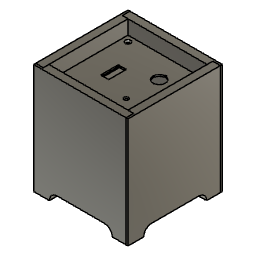
box (Autodesk Fusion 360 design; units mm, degrees)
Autodesk Fusion 360 part; units mm, degrees
sketch "base sketch" plane through (0, 0, 0) normal (0, 0, 1) x (1, 0, 0)
  line L0 (76.2, 76.2) -> (-76.2, 76.2)
  line L1 (-76.2, 76.2) -> (-76.2, -76.2)
  line L2 (-76.2, -76.2) -> (76.2, -76.2)
  line L3 (76.2, -76.2) -> (76.2, 76.2)
  line L4 (76.2, 76.2) -> (-76.2, -76.2) construction
  line L5 (-76.2, 76.2) -> (76.2, -76.2) construction
  line L6 (-76.2, -73.025) -> (-63.9, -73.025)
  line L7 (-63.9, -73.025) -> (-63.9, -63.9)
  line L8 (-63.9, -63.9) -> (73.025, -63.9)
  line L9 (73.025, -63.9) -> (73.025, -76.2)
  dimension "d1" = 152.4
  dimension "d2" = 152.4
  dimension "ply" = 12.3
  dimension "d4" = 12.3
  dimension "outside_radius" = 3.175
  dimension "d6" = 3.175
  constraint horizontal L0
  constraint perpendicular L0 L1
  constraint parallel L0 L2
  constraint parallel L1 L3
  constraint coincident L4 origin
  constraint coincident L5 origin
  constraint coincident L1 L6.start
  constraint perpendicular L1 L6
  constraint perpendicular L6 L7
  constraint coincident L2 L9.end
  constraint perpendicular L2 L9
  constraint horizontal L8
  measures "d1" distance of L1.end L2.end
  measures "d2" distance of L0.end L1.end
  measures "ply" distance of L2 L8
  measures "d4" distance of L1 L7
  measures "outside_radius" distance of L2 L6
  measures "d6" distance of L3 L9
extrude "Extrude1" add sketch "base sketch" along normal blind 177.8 contours L1 L2 L6 L7 L8 L9 makes body 1 in component "side"
sketch "bottom gap" plane through (0, -76.2, 0) normal (0, -1, 0) x (1, 0, 0) in component "side"
  line L0 (-76.2, 0) -> (73.025, 0)
  line L1 (73.025, 0) -> (73.025, 177.8)
  line L2 (73.025, 177.8) -> (-76.2, 177.8)
  line L3 (-76.2, 177.8) -> (-76.2, 0)
  line L4 (-76.2, 0) -> (-78.2761, 0) construction
  line L5 (76.2, 0) -> (-76.2, 0)
  line L6 (76.2, 0) -> (-76.2, 0) construction
  line L7 (0, 0) -> (0, 12.7) construction
  line L8 (-38.1, 12.7) -> (38.1, 12.7)
  arc A0 (-38.1, 12.7) -> (-50.8, 0) centre (-38.1, 0) ccw
  line L9 (-76.2, 0) -> (76.2, 0)
  arc A1 (50.8, 0) -> (38.1, 12.7) centre (38.1, 0) ccw
  point P0 (76.2, 0)
  dimension "d9" = 12.7
  dimension "d10" = 25.4
  dimension "d12" = 25.4
  constraint coincident L0.start L3.end
  constraint coincident P0 L5.start
  constraint coincident L7.start origin
  constraint perpendicular L5 L7
  constraint horizontal L8
  constraint coincident L7.end L8
  constraint coincident L5 A0.centre
  constraint tangent L8 A0
  constraint coincident A0.end L9
  constraint coincident L9 A1.start
  constraint coincident L5 A1.centre
  constraint coincident L8.end A1.end
  constraint tangent L8 A1
  measures "d9" distance of L6 L8
  measures "d10" distance of L0.start A0.end
  measures "d12" distance of P0 A1.start
extrude "Extrude2" cut sketch "bottom gap" against normal up to surface (12.3 mm away) contours L0 L5 L8 A0 L9 A1 bodies 1 in component "side"
component_pattern "component pattern"
ref_plane "WorkPlane1" through (0, 0, 25.4) normal (0, 0, 1) x (1, 0, 0)
sketch "Sketch3" plane through (0, 0, 25.4) normal (0, 0, 1) x (1, 0, 0)
  circle A0 centre (55.4048, 55.4048) radius 6.1
  line L0 (76.2, 76.2) -> (-76.2, -76.2)
  line L1 (-73.025, 63.9) -> (63.9, 63.9) construction
  line L2 (63.9, 73.025) -> (63.9, -63.9) construction
  line L3 (-63.9, -73.025) -> (-63.9, 63.9)
  line L4 (-38.1, 63.9) -> (38.1, 63.9)
  line L5 (76.2, 73.025) -> (76.2, 76.2)
  line L6 (76.2, 76.2) -> (-73.025, 76.2)
  line L7 (-73.025, 76.2) -> (-73.025, 63.9)
  line L8 (-73.025, 63.9) -> (63.9, 63.9)
  line L9 (63.9, 63.9) -> (63.9, 73.025)
  line L10 (63.9, 73.025) -> (76.2, 73.025)
  line L11 (-73.025, 76.2) -> (-76.2, 76.2)
  line L12 (-76.2, 76.2) -> (-76.2, -73.025)
  line L13 (-76.2, -73.025) -> (-63.9, -73.025)
  line L14 (-63.9, -73.025) -> (-63.9, 63.9)
  line L15 (-63.9, 63.9) -> (-73.025, 63.9)
  line L16 (-73.025, 63.9) -> (-73.025, 76.2)
  line L17 (-76.2, -73.025) -> (-76.2, -76.2)
  line L18 (-76.2, -76.2) -> (73.025, -76.2)
  line L19 (73.025, -76.2) -> (73.025, -63.9)
  line L20 (73.025, -63.9) -> (-63.9, -63.9)
  line L21 (-63.9, -63.9) -> (-63.9, -73.025)
  line L22 (-63.9, -73.025) -> (-76.2, -73.025)
  line L23 (73.025, -76.2) -> (76.2, -76.2)
  line L24 (76.2, -76.2) -> (76.2, 73.025)
  line L25 (76.2, 73.025) -> (63.9, 73.025)
  line L26 (63.9, 73.025) -> (63.9, -63.9)
  line L27 (63.9, -63.9) -> (73.025, -63.9)
  line L28 (73.025, -63.9) -> (73.025, -76.2)
  line L29 (-68, 68) -> (68, 68)
  line L30 (68, 68) -> (68, -68)
  line L31 (68, -68) -> (-68, -68)
  line L32 (-68, -68) -> (-68, 68)
  line L33 (-63.9, -63.9) -> (73.025, -63.9)
  line L34 (61.85, 36.85) -> (61.85, -36.85)
  line L35 (36.85, -61.85) -> (-36.85, -61.85)
  line L36 (-61.85, -36.85) -> (-61.85, 36.85)
  line L37 (-36.85, 61.85) -> (36.85, 61.85)
  line L38 (-36.85, -61.85) -> (-61.85, -36.85)
  line L39 (61.85, -36.85) -> (36.85, -61.85)
  line L40 (-61.85, 36.85) -> (-36.85, 61.85)
  line L41 (61.85, 36.85) -> (36.85, 61.85)
  point P0 (61.85, 61.85)
  point P1 (61.85, -61.85)
  point P2 (-61.85, -61.85)
  point P3 (-61.85, 61.85)
  dimension "d18" = 12.2
  dimension "d27" = 4.1
  dimension "d28" = 4.1
  dimension "d29" = 4.1
  dimension "d30" = 4.1
  dimension "d32" = 25
  dimension "d33" = 25
  dimension "d34" = 25
  dimension "d35" = 25
  dimension "d36" = 25
  dimension "d37" = 25
  dimension "d38" = 25
  dimension "d39" = 25
  constraint coincident A0.centre L0
  constraint horizontal L29
  constraint vertical L30
  constraint horizontal L31
  constraint vertical L32
  constraint coincident P2 L35
  constraint coincident P2 L36
  constraint coincident P1 L34
  constraint coincident P1 L35
  constraint coincident P3 L36
  constraint coincident P3 L37
  constraint coincident P0 L34
  constraint coincident P0 L37
  measures "d18" diameter of A0
  measures "d27" distance of L8 L29
  measures "d28" distance of L14 L32
  measures "d29" distance of L31 L33
  measures "d30" distance of L26 L30
  measures "d32" distance of P2 L35.end
  measures "d33" distance of P2 L36.start
  measures "d34" distance of P1 L34.end
  measures "d35" distance of P1 L35.start
  measures "d36" distance of P3 L36.end
  measures "d37" distance of P3 L37.start
  measures "d38" distance of P0 L34.start
  measures "d39" distance of P0 L37.end
extrude "Extrude1'" add sketch "Sketch3" along normal blind 12.3 separate body contours A0 L0 | A0 L0 L20 L26 L33 L34 L35 L38 L39 L41 | A0 L0 | A0 L0 L3 L4 L8 L14 L36 L37 L38 L40 L41 | L0 L9 L26 L29 | L4 L8 L9 L15 L26 L29 L32 | L0 L20 L26 L27 L30 L33 | L3 L14 L20 L21 L27 L30 L31 L33 | L0 L3 L14 L21 L31 | L0 L3 L8 L14 L15 L32 makes body 2 in component "bottom"
sketch "Sketch1" plane through (73.025, 0, 0) normal (1, 0, 0) x (0, 1, 0) in component "side"
  line L0 (-76.2, 0) -> (-63.9, 0)
  line L1 (-63.9, 0) -> (-63.9, 177.8)
  line L2 (-63.9, 177.8) -> (-76.2, 177.8)
  line L3 (-76.2, 177.8) -> (-76.2, 0)
  line L4 (-68, 25.4) -> (68, 25.4)
  line L5 (68, 25.4) -> (68, 37.7)
  line L6 (68, 37.7) -> (-68, 37.7)
  line L7 (-68, 37.7) -> (-68, 25.4)
  line L8 (-68, 140.4) -> (68, 140.4)
  line L9 (68, 140.4) -> (68, 152.7)
  line L10 (68, 152.7) -> (-68, 152.7)
  line L11 (-68, 152.7) -> (-68, 140.4)
extrude "Extrude3" cut sketch "Sketch1" against normal up to surface (136.925 mm away) contours L1 L4 L6 L7 | L1 L8 L10 L11 bodies 1 in component "side"
extrude "Extrude1''" add sketch "Sketch3" along normal blind 12.3 separate body contours A0 L0 | A0 L0 L20 L26 L33 L34 L35 L38 L39 L41 | A0 L0 | A0 L0 L3 L4 L8 L14 L36 L37 L38 L40 L41 | L0 L9 L26 L29 | L4 L8 L9 L15 L26 L29 L32 | L0 L20 L26 L27 L30 L33 | L3 L14 L20 L21 L27 L30 L31 L33 | L0 L3 L14 L21 L31 | L0 L3 L8 L14 L15 L32 makes body 3 in component "top"
extrude "Extrude2'" cut sketch "Sketch3" along normal blind 2.75 contours A0 L0 | A0 L0 bodies 2 in component "bottom"
pattern_circular "C-Pattern1" count 4 over 360 about axis through (0, 0, 1.75) along (0, 0, 1) of "Extrude2'" in component "bottom"
extrude "Extrude1'''" add sketch "base sketch" along normal blind 177.8 separate body contours L1 L2 L6 L7 L8 L9 makes body 4 in component "side sensor"
sketch "bottom gap (2)" plane through (0, -76.2, 0) normal (0, -1, 0) x (1, 0, 0) in component "side sensor"
  line L0 (-76.2, 0) -> (73.025, 0)
  line L1 (73.025, 0) -> (73.025, 177.8)
  line L2 (73.025, 177.8) -> (-76.2, 177.8)
  line L3 (-76.2, 177.8) -> (-76.2, 0)
  line L4 (-76.2, 0) -> (-78.2761, 0) construction
  line L5 (76.2, 0) -> (-76.2, 0)
  line L6 (76.2, 0) -> (-76.2, 0) construction
  line L7 (0, 0) -> (0, 12.7) construction
  line L8 (-38.1, 12.7) -> (38.1, 12.7)
  arc A0 (-38.1, 12.7) -> (-50.8, 0) centre (-38.1, 0) ccw
  line L9 (-76.2, 0) -> (76.2, 0)
  arc A1 (50.8, 0) -> (38.1, 12.7) centre (38.1, 0) ccw
  point P0 (76.2, 0)
  dimension "d9_1" = 12.7
  dimension "d10_1" = 25.4
  dimension "d12_1" = 25.4
  constraint coincident L0.start L3.end
  constraint coincident P0 L5.start
  constraint coincident L7.start origin
  constraint perpendicular L5 L7
  constraint horizontal L8
  constraint coincident L7.end L8
  constraint coincident L5 A0.centre
  constraint tangent L8 A0
  constraint coincident A0.end L9
  constraint coincident L9 A1.start
  constraint coincident L5 A1.centre
  constraint coincident L8.end A1.end
  constraint tangent L8 A1
  measures "d9_1" distance of L6 L8
  measures "d10_1" distance of L0.start A0.end
  measures "d12_1" distance of P0 A1.start
extrude "Extrude2''" cut sketch "bottom gap (2)" against normal up to surface (12.3 mm away) contours L0 L5 L8 A0 L9 A1 bodies 4 in component "side sensor"
sketch "Sketch1 (2)" plane through (73.025, 0, 0) normal (1, 0, 0) x (0, 1, 0) in component "side sensor"
  line L0 (-76.2, 0) -> (-63.9, 0)
  line L1 (-63.9, 0) -> (-63.9, 177.8)
  line L2 (-63.9, 177.8) -> (-76.2, 177.8)
  line L3 (-76.2, 177.8) -> (-76.2, 0)
  line L4 (-68, 25.4) -> (68, 25.4)
  line L5 (68, 25.4) -> (68, 37.7)
  line L6 (68, 37.7) -> (-68, 37.7)
  line L7 (-68, 37.7) -> (-68, 25.4)
  line L8 (-68, 140.4) -> (68, 140.4)
  line L9 (68, 140.4) -> (68, 152.7)
  line L10 (68, 152.7) -> (-68, 152.7)
  line L11 (-68, 152.7) -> (-68, 140.4)
extrude "Extrude3'" cut sketch "Sketch1 (2)" against normal up to surface (136.925 mm away) contours L1 L4 L6 L7 | L1 L8 L10 L11 bodies 4 in component "side sensor"
sketch "sensor" plane through (-76.2, 0, 0) normal (-1, 0, 0) x (0, -1, 0)
  arc A0 (50.8, 0) -> (38.1, 12.7) centre (38.1, 0) ccw
  line L0 (50.8, 0) -> (73.025, 0)
  line L1 (73.025, 0) -> (73.025, 177.8)
  line L2 (73.025, 177.8) -> (-76.2, 177.8)
  line L3 (-76.2, 177.8) -> (-76.2, 0)
  line L4 (-76.2, 0) -> (-50.8, 0)
  arc A1 (-38.1, 12.7) -> (-50.8, 0) centre (-38.1, 0) ccw
  line L5 (-38.1, 12.7) -> (38.1, 12.7)
  line L6 (76.2, 0) -> (76.2, 177.8) construction
  line L7 (76.2, 127) -> (-76.2, 127) construction
  line L8 (0, 127) -> (0, 102.1177) construction
  circle A2 centre (-13, 127) radius 8
  circle A3 centre (13, 127) radius 8
  dimension "d48" = 127
  dimension "d49" = 26
  dimension "d50" = 16
  constraint coincident L6 L7.start
  constraint coincident L3 L7.end
  constraint perpendicular L3 L7
  constraint midpoint L7 L8.start
  constraint perpendicular L7 L8
  constraint coincident L7 A2.centre
  constraint coincident L7 A3.centre
  constraint equal A2 A3
  constraint symmetric L8 A2.centre A3.centre
  measures "d48" distance of L0 L7
  measures "d49" distance of A2.centre A3.centre
  measures "d50" diameter of A2
extrude "Extrude4" cut sketch "sensor" against normal up to surface (12.3 mm away) contours A2 | A3 sketch seen with x (0, 1, 0) y (-1, 0, 0) z (0, 0, 1) at (0, 0, 0) bodies 4 in component "side sensor"
sketch "Sketch1 (3)" plane through (0, 0, 25.4) normal (0, 0, -1) x (1, 0, 0) in component "bottom cover"
  circle A0 centre (55.4048, 55.4048) radius 6.1
  circle A1 centre (-55.4048, 55.4048) radius 6.1
  circle A2 centre (-55.4048, -55.4048) radius 6.1
  circle A3 centre (55.4048, -55.4048) radius 6.1
  line L0 (61.85, 36.85) -> (61.85, -36.85)
  line L1 (61.85, -36.85) -> (36.85, -61.85)
  line L2 (36.85, -61.85) -> (-36.85, -61.85)
  line L3 (-36.85, -61.85) -> (-61.85, -36.85)
  line L4 (-61.85, -36.85) -> (-61.85, 36.85)
  line L5 (-61.85, 36.85) -> (-36.85, 61.85)
  line L6 (-36.85, 61.85) -> (36.85, 61.85)
  line L7 (36.85, 61.85) -> (61.85, 36.85)
  line L8 (68, 68) -> (-68, 68)
  line L9 (-68, 68) -> (-68, -68)
  line L10 (-68, -68) -> (68, -68)
  line L11 (68, -68) -> (68, 68)
  line L12 (-62.9, 62.9) -> (62.9, 62.9)
  line L13 (62.9, 62.9) -> (62.9, -62.9)
  line L14 (62.9, -62.9) -> (-62.9, -62.9)
  line L15 (-62.9, -62.9) -> (-62.9, 62.9)
  line L16 (63.9, -38.1) -> (63.9, 38.1)
  line L17 (38.1, 63.9) -> (-38.1, 63.9)
  line L18 (-63.9, 38.1) -> (-63.9, -38.1)
  line L19 (-38.1, -63.9) -> (38.1, -63.9)
  line L20 (0, 0) -> (47.1189, 0) construction
  line L21 (0, 0) -> (0, 34.7733) construction
  circle A4 centre (10, 0) radius 11
  circle A5 centre (-10, 0) radius 11
  line L22 (-10, 11) -> (10, 11)
  line L23 (10, -11) -> (-10, -11)
  line L24 (0, 0) -> (-38.8885, 0) construction
  line L25 (-10, 11) -> (-10, -11)
  line L26 (10, -11) -> (10, 11)
  dimension "d53" = 1
  dimension "d54" = 1
  dimension "d55" = 1
  dimension "d56" = 1
  dimension "d57" = 22
  dimension "d58" = 22
  dimension "d59" = 20
  constraint horizontal L12
  constraint vertical L13
  constraint horizontal L14
  constraint vertical L15
  constraint coincident L20.start L21.start
  constraint horizontal L20
  constraint perpendicular L20 L21
  constraint coincident L20 A4.centre
  constraint coincident A5 L22.start
  constraint coincident A4 L22.end
  constraint tangent A4 L22
  constraint coincident A4 L23.start
  constraint coincident A5 L23.end
  constraint tangent A5 L23
  constraint tangent A4 L23
  constraint tangent A5 L22
  constraint perpendicular L21 L24
  constraint coincident A5.centre L24
  constraint symmetric L21 A4.centre A5.centre
  measures "d53" distance of L13 L16
  measures "d54" distance of L12 L17
  measures "d55" distance of L15 L18
  measures "d56" distance of L14 L19
  measures "d57" diameter of A4
  measures "d58" diameter of A5
  measures "d59" distance of L25 L26
extrude "Extrude1''''" add sketch "Sketch1 (3)" along normal blind 5 separate body contours A0 | A1 | A2 | A3 | L0 L1 L2 L3 L4 L5 L6 L7 | L12 L13 L14 L15 | A4 L26 | A4 A5 L26 | A4 A5 L22 | A4 A5 L23 | A4 A5 | A4 A5 L25 | A5 L25 makes body 5 in component "bottom cover"
extrude "Extrude2'''" cut sketch "Sketch1 (3)" along normal blind 2.7 contours A0 | A1 | A2 | A3 | L0 L1 L2 L3 L4 L5 L6 L7 | A4 L26 | A4 A5 L26 | A4 A5 L22 | A4 A5 L23 | A4 A5 | A4 A5 L25 | A5 L25 bodies 5 in component "bottom cover"
extrude "Extrude1'''''" [suppressed]
extrude "Extrude3''" cut sketch "Sketch1 (3)" along normal blind 30 contours A4 L26 | A5 L25 bodies 5 in component "bottom cover"
extrude "Extrude4'" add sketch "Sketch1 (3)" against normal blind 3 from surface at 2.7 contours A4 A5 L26 | A4 A5 L22 | A4 A5 L23 | A4 A5 | A4 A5 L25 bodies 5 in component "bottom cover"
sketch "Sketch2" plane through (0, 0, 37.7) normal (0, 0, 1) x (-1, 0, 0) in component "top"
  line L0 (-61.85, -36.85) -> (-61.85, 36.85)
  line L1 (-61.85, 36.85) -> (-36.85, 61.85)
  line L2 (-36.85, 61.85) -> (36.85, 61.85)
  line L3 (36.85, 61.85) -> (61.85, 36.85)
  line L4 (61.85, 36.85) -> (61.85, -36.85)
  line L5 (61.85, -36.85) -> (36.85, -61.85)
  line L6 (36.85, -61.85) -> (-36.85, -61.85)
  line L7 (-36.85, -61.85) -> (-61.85, -36.85)
  line L8 (68, 68) -> (-68, 68)
  line L9 (-68, 68) -> (-68, -68)
  line L10 (-68, -68) -> (68, -68)
  line L11 (68, -68) -> (68, 68)
  line L12 (62.9, -62.9) -> (62.9, 62.9) construction
  line L13 (-62.9, -62.9) -> (62.9, -62.9) construction
  line L14 (-62.9, 62.9) -> (-62.9, -62.9) construction
  line L15 (62.9, 62.9) -> (-62.9, 62.9) construction
  line L16 (-61.85, 36.85) -> (-36.85, 61.85)
  line L17 (-36.85, -61.85) -> (-61.85, -36.85)
  line L18 (61.85, -36.85) -> (36.85, -61.85)
  line L19 (36.85, 61.85) -> (61.85, 36.85)
  line L20 (62.9, 62.9) -> (49.35, 49.35) construction
  line L21 (-63.65, -63.65) -> (63.65, -63.65)
  line L22 (63.65, -63.65) -> (63.65, 63.65)
  line L23 (63.65, 63.65) -> (-63.65, 63.65)
  line L24 (-63.65, 63.65) -> (-63.65, -63.65)
  point P0 (54.2997, 54.2997)
  dimension "d71" = 7
  dimension "d72" = 0.75
  constraint coincident L12.end L15.start
  constraint midpoint L19 L20.end
  constraint coincident L20 P0
  measures "d71" distance of L20.end P0
extrude "Extrude1''''''" add sketch "Sketch2" along normal blind 2.5 separate body contours L0 L1 L2 L3 L4 L5 L6 L7 L16 L17 L18 L19 | L21 L22 L23 L24 sketch seen with x (1, 0, 0) y (0, 1, 0) z (0, 0, 1) at (0, 0, 115) makes body 6 in component "top cover"
sketch "Sketch1 (4)" plane through (0, 0, 155.2) normal (0, 0, 1) x (-1, 0, 0) in component "top cover"
  line L0 (-63.65, 63.65) -> (-63.65, -63.65)
  line L1 (-63.65, -63.65) -> (63.65, -63.65)
  line L2 (63.65, -63.65) -> (63.65, 63.65)
  line L3 (63.65, 63.65) -> (-63.65, 63.65)
  point P0 (54.2997, 54.2997)
hole "Hole1" at (-54.2997, -54.2997, 155.2) direction (0, 0, -1) diameter 4.5 depth 10 tip angle 180 countersink diameter 9 countersink angle 90 bodies 6 in component "top cover"
pattern_circular "C-Pattern1'" count 4 over 360 about axis through (0, 0, 1.75) along (0, 0, 1) of "Hole1" in component "top cover"
sketch "Sketch2 (2)" plane through (0, 0, 155.2) normal (0, 0, 1) x (-1, 0, 0) in component "top cover"
  circle A0 centre (54.2997, -54.2997) radius 4.5
  circle A1 centre (-54.2997, -54.2997) radius 4.5
  circle A2 centre (-54.2997, 54.2997) radius 4.5
  circle A3 centre (54.2997, 54.2997) radius 4.5
  line L0 (-63.65, 63.65) -> (-63.65, -63.65)
  line L1 (-63.65, -63.65) -> (63.65, -63.65)
  line L2 (63.65, -63.65) -> (63.65, 63.65)
  line L3 (63.65, 63.65) -> (-63.65, 63.65)
  line L4 (28.7361, 13) -> (18.2361, 13)
  line L5 (18.2361, 13) -> (18.2361, -13)
  line L6 (18.2361, -13) -> (28.7361, -13)
  line L7 (28.7361, -13) -> (28.7361, 13)
  circle A4 centre (-23.7665, 26.567) radius 3.6
  circle A5 centre (-23.7665, -26.567) radius 10
  line L8 (0, 0) -> (54.4333, 0) construction
  circle A6 centre (-23.7665, 26.567) radius 7.5
  line L9 (-23.7665, 26.567) -> (-23.7665, -26.567) construction
  line L10 (29.7361, 19.5) -> (17.2361, 19.5)
  line L11 (17.2361, 19.5) -> (17.2361, -20.5)
  line L12 (17.2361, -20.5) -> (29.7361, -20.5)
  line L13 (29.7361, -20.5) -> (29.7361, 19.5)
  line L14 (23.4861, 13) -> (23.4861, -13) construction
  line L15 (-23.7665, -26.567) -> (-23.7665, -37.6539) construction
  line L16 (-22.2665, -36.4539) -> (-22.2665, -37.6539)
  line L17 (-22.2665, -37.6539) -> (-25.2665, -37.6539)
  line L18 (-25.2665, -37.6539) -> (-25.2665, -36.4539)
  dimension "d82" = 26
  dimension "d83" = 10.5
  dimension "d84" = 7.2
  dimension "d85" = 15
  dimension "d86" = 20
  dimension "d87" = 12.5
  dimension "d88" = 40
  dimension "d89" = 6.5
  dimension "d90" = 1.2
  dimension "d91" = 3
  constraint horizontal L4
  constraint vertical L5
  constraint horizontal L6
  constraint vertical L7
  constraint coincident L8.start origin
  constraint perpendicular L7 L8
  constraint symmetric L4 L6 L8
  constraint concentric A4 A6
  constraint coincident A4.centre A6.centre
  constraint coincident A5.centre L9.end
  constraint vertical L9
  constraint symmetric A5.centre L8 A4.centre
  constraint horizontal L10
  constraint vertical L11
  constraint horizontal L12
  constraint vertical L13
  constraint midpoint L4 L14.start
  constraint midpoint L6 L14.end
  constraint symmetric L11 L13 L14
  constraint parallel L9 L15
  constraint coincident A5 L16.start
  constraint vertical L16
  constraint perpendicular L15 L17
  constraint coincident A5 L18.end
  constraint perpendicular L17 L18
  constraint coincident L15.end L17
  measures "d82" distance of L4 L6
  measures "d83" distance of L5 L7
  measures "d84" diameter of A4
  measures "d85" diameter of A6
  measures "d86" diameter of A5
  measures "d87" distance of L11 L13
  measures "d88" distance of L10 L12
  measures "d89" distance of L4 L10
  measures "d90" distance of L16.start L16.end
  measures "d91" distance of L16.end L17.end
extrude "Extrude2''''" cut sketch "Sketch2 (2)" against normal blind 10 contours L4 L5 L6 L7 | A4 | A5 | A5 L16 L17 L18 bodies 6 in component "top cover"
chamfer "Chamfer1" distance 1.25 angle 45 4 edges at (-28.7361, 0, 155.2) (-23.4861, -13, 155.2) (-18.2361, 0, 155.2) (-23.4861, 13, 155.2) on bodies 6 in component "top cover"
extrude "Extrude3'''" cut sketch "Sketch2 (2)" along normal blind 1 from surface at -2.5 contours L10 L11 L12 L13 bodies 6 in component "top cover"
sketch "Sketch3 (2)" plane through (0, 0, 152.7) normal (0, 0, -1) x (1, 0, 0) in component "top cover"
  line L0 (-29.7361, -20.5) -> (-29.7361, 19.5)
  line L1 (-29.7361, 19.5) -> (-17.2361, 19.5)
  line L2 (-17.2361, 19.5) -> (-17.2361, -20.5)
  line L3 (-17.2361, -20.5) -> (-29.7361, -20.5)
  circle A0 centre (23.7665, 26.567) radius 3.6
  line L4 (25.2665, -36.4539) -> (25.2665, -37.6539)
  line L5 (25.2665, -37.6539) -> (22.2665, -37.6539)
  line L6 (22.2665, -37.6539) -> (22.2665, -36.4539)
  arc A1 (25.2665, -36.4539) -> (22.2665, -36.4539) centre (23.7665, -26.567) ccw
  circle A2 centre (-54.2997, -54.2997) radius 2.25
  circle A3 centre (54.2997, -54.2997) radius 2.25
  circle A4 centre (54.2997, 54.2997) radius 2.25
  circle A5 centre (-54.2997, 54.2997) radius 2.25
  line L7 (63.65, -63.65) -> (63.65, 63.65)
  line L8 (63.65, 63.65) -> (-63.65, 63.65)
  line L9 (-63.65, 63.65) -> (-63.65, -63.65)
  line L10 (-63.65, -63.65) -> (63.65, -63.65)
  line L11 (-31.7361, -22.5) -> (-31.7361, 21.5)
  line L12 (-31.7361, 21.5) -> (-15.2361, 21.5)
  line L13 (-15.2361, 21.5) -> (-15.2361, -22.5)
  line L14 (-15.2361, -22.5) -> (-31.7361, -22.5)
  dimension "d98" = -2
extrude "Extrude4''" add sketch "Sketch3 (2)" along normal blind 2 contours L11 L12 L13 L14 bodies 6 in component "top cover"
component "side" placed x (1, 0, 0) y (0, 1, 0) z (0, 0, 1) at (0, 0, 0)
component "side" placed x (0, 1, 0) y (-1, 0, 0) z (0, 0, 1) at (0, 0, 0)
component "side" placed x (-1, 0, 0) y (0, -1, 0) z (0, 0, 1) at (0, 0, 0)
component "bottom" placed x (1, 0, 0) y (0, 1, 0) z (0, 0, 1) at (0, 0, 0)
component "top" placed x (1, 0, 0) y (0, 1, 0) z (0, 0, 1) at (0, 0, 115)
component "side sensor" placed x (0, -1, 0) y (1, 0, 0) z (0, 0, 1) at (0, 0, 0)
component "bottom cover" placed x (1, 0, 0) y (0, 1, 0) z (0, 0, 1) at (0, 0, 0)
component "top cover" placed x (1, 0, 0) y (0, 1, 0) z (0, 0, 1) at (0, 0, 0)
equation "d4 = ply"
equation "outside_radius = 1 / 8 * 1 in"
equation "d6 = outside_radius"
equation "d27 = ply / 3"
equation "d28 = ply / 3"
equation "d29 = ply / 3"
equation "d30 = ply / 3"
equation "d33 = d32"
equation "d35 = d34"
equation "d37 = d36"
equation "d39 = d38"
equation "d40 = ply"
equation "d40_1 = ply"
